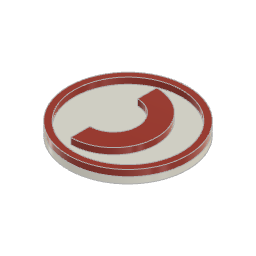
_C.475d76b7-dd14-4272-ae3d-81a79d86ffa4 (Autodesk Fusion 360 design; units mm, degrees)
Autodesk Fusion 360 part; units mm, degrees
sketch "Sketch1" plane through (0, 0, 0) normal (0, 0, 1) x (1, 0, 0)
  circle A0 centre (0, 0) radius 15.875
  circle A1 centre (0, 0) radius 14.2875
  line L0 (0, 0) -> (-3.81, 0)
  circle A2 centre (-3.81, 0) radius 6.35
  circle A3 centre (-3.81, 0) radius 11.43
  line L1 (-3.81, 0) -> (-3.81, 11.43)
  line L2 (-3.81, 0) -> (-3.81, -11.43)
  dimension "d16" = 3.81
  dimension "d17" = 12.7
  dimension "d18" = 22.86
  constraint coincident A0.centre A1.centre
  constraint horizontal L0
  constraint coincident L0.end A2.centre
  constraint concentric A2 A3
  constraint coincident A3 L1.end
  constraint perpendicular L0 L1
  constraint coincident A3 L2.end
  constraint perpendicular L0 L2
  measures "d16" distance of A0.centre L0.end
  measures "d17" diameter of A2
  measures "d18" diameter of A3
extrude "Extrude1" add sketch "Sketch1" against normal blind 1 contours A0 | A1 A3 | A1 A2 A3 L1 L2 | A1 A3 | A2 A3 L1 L2 | A2 L1 L2 | A2 L1 L2 makes body 1 in component "Base"
extrude "Extrude1'" add sketch "Sketch1" along normal blind 1 separate body contours A0 | A1 A3 | A2 A3 L1 L2 picked at (-14.5817, 0) makes body 2 at (15.2335, -1.4985, 0) makes body 3 at (-1.4952, 9.4308, 0) in component "Top"
scale "Scale1" factors (0.6, 0.6, 1) about (-3.81, -6.35, 0) bodies 2 3 in component "Top"
scale "Scale1'" factors (0.6, 0.6, 1) about (-3.81, -6.35, 0) bodies 1 in component "Base"
component "Base" placed x (1, 0, 0) y (0, 1, 0) z (0, 0, 1) at (0, 0, 0)
component "Top" placed x (1, 0, 0) y (0, 1, 0) z (0, 0, 1) at (0, 0, 0)
